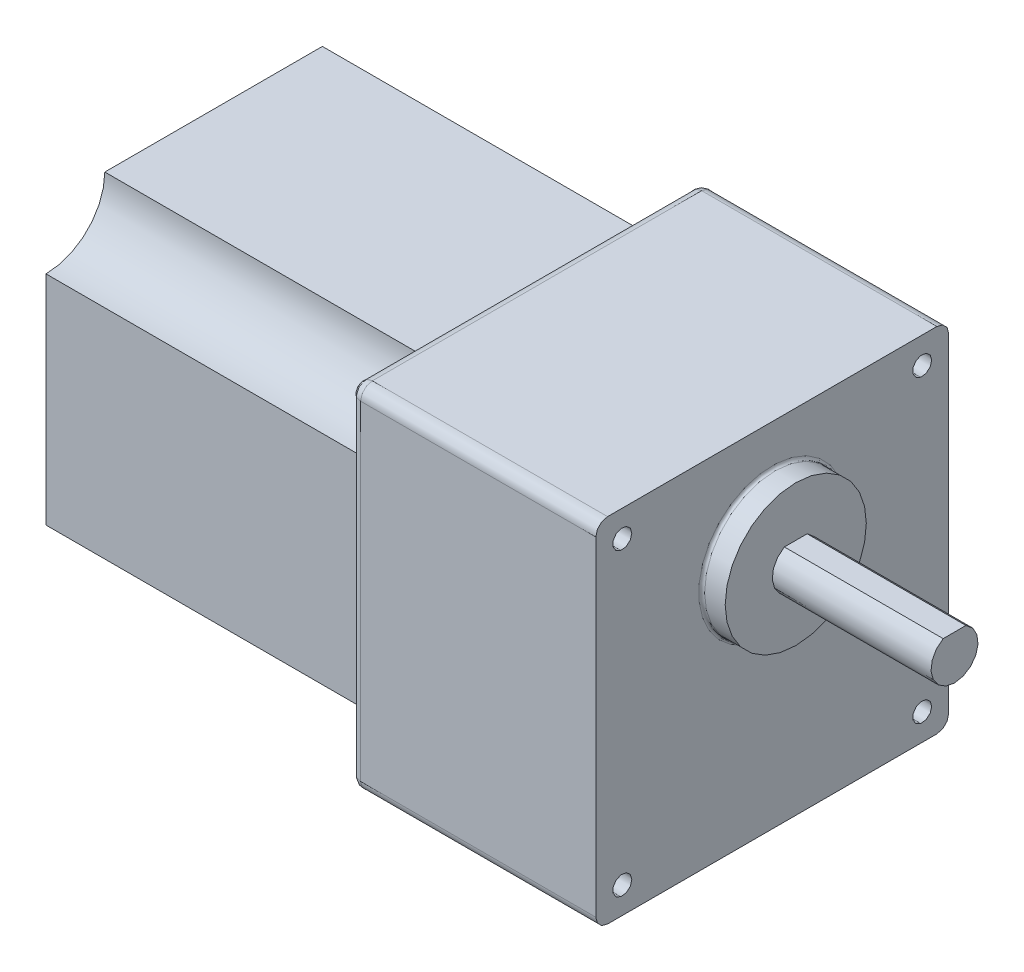
# Autodesk Inventor part: MOTOR MODEL
Saved by Autodesk Inventor 2023 (Build 270158000, 158)
## iProperties
Created: 2022-09-15
Part Number: MOTOR MODEL
Material: Acetal Resin, Black
Document SubType Name: Modeling
Designer: D.C. Eksteen
Density: 1.425 g/cm^3
Appearance: Smooth - Black
Author: D.C. Eksteen
Autodesk Inventor part; units mm, degrees
ref_plane "YZ Plane" through (0, 0, 0) normal (1, 0, 0) x (0, 1, 0)
ref_plane "XZ Plane" through (0, 0, 0) normal (0, 1, 0) x (-1, 0, 0)
ref_plane "XY Plane" through (0, 0, 0) normal (0, 0, 1) x (1, 0, 0)
sketch "Sketch1" plane through (0, 0, 0) normal (1, 0, 0) x (0, 1, 0)
  line L0 (0, 0) -> (60, 0)
  line L1 (60, 0) -> (60, -60)
  line L2 (60, -60) -> (0, -60)
  line L3 (0, -60) -> (0, 0)
  dimension "d0" = 60
  dimension "d1" = 60
  constraints: 8 end point, 2 parallel, 1 horizontal, 1 perpendicular
  measures "d0" distance of L1.end L2.end
  measures "d1" distance of L0.end L1.end
extrude "Extrusion1" add sketch "Sketch1" against normal blind 42
sketch "Sketch2" plane through (-42, 0, 0) normal (-1, 0, 0) x (0, 0, 1)
  line L0 (-60, 60) -> (-60, 0) projected
  line L1 (-60, 0) -> (0, 0) projected
  line L2 (0, 0) -> (0, 60) projected
  line L3 (0, 60) -> (-60, 60) projected
  line L4 (-58.5, 58.5) -> (-58.5, 1.5)
  line L5 (-58.5, 1.5) -> (-1.5, 1.5)
  line L6 (-1.5, 1.5) -> (-1.5, 58.5)
  line L7 (-1.5, 58.5) -> (-58.5, 58.5)
  dimension "d4" = 1.5
  constraints: 8 end point, 3 other
  measures "d4" distance between parallel lines of L3 L7
extrude "Extrusion2" add sketch "Sketch2" along normal blind 53 contours L7 L6 L5 L4
sketch "Sketch3" plane through (0, 0, 0) normal (1, 0, 0) x (0, 0, -1)
  line L0 (60, 0) -> (60, 60) projected
  line L1 (60, 60) -> (0, 60) projected
  line L2 (0, 60) -> (0, 0) projected
  line L3 (0, 0) -> (60, 0) projected
  circle A0 centre (30, 41) radius 12
  dimension "d8" = 24
  dimension "d9" = 19
  dimension "d10" = 30
  constraints: 1 centre point
  measures "d8" diameter of A0
  measures "d9" distance from line of L1 A0.centre
  measures "d10" distance from line of L2 A0.centre
extrude "Extrusion3" add sketch "Sketch3" along normal blind 4 contours A0
sketch "Sketch4" plane through (4, 41, -30) normal (1, 0, 0) x (0, 0, -1)
  circle A0 centre (0, 0) radius 12 projected
  circle A1 centre (0, 0) radius 4
  line L0 (-1.9365, 3.5) -> (1.9365, 3.5)
  point P0 (-30, -41)
  dimension "d13" = 8
  dimension "d16" = 3.5
  constraints: 2 end point, 2 point on circle, 1 centre point, 1 coincident, 1 horizontal
  measures "d13" diameter of A1
  measures "d16" distance from line of L0 A1.centre
extrude "Extrusion4" add sketch "Sketch4" along normal blind 27 contours A1 L0 picked at (0.0805, 0.6484)
sketch "Sketch5" plane through (0, 0, 0) normal (1, 0, 0) x (0, 0, -1)
  point P0 (0, 0)
sketch "Sketch6" plane through (-95, 0, 0) normal (-1, 0, 0) x (0, 0, 1)
  point P0 (0, 0)
fillet "Fillet2" radius 10 4 edges at (-68.5, 58.5, -58.5) (-68.5, 1.5, -58.5) (-68.5, 1.5, -1.5) (-68.5, 58.5, -1.5) inverted yes
fillet "Fillet3" radius 2 8 edges at (-42, 30, -60) (-42, 60, -30) (-21, 60, -60) (-42, 0, -30) (-21, 0, -60) (-21, 60, 0) (-42, 30, 0) (-21, 0, 0)
fillet "Fillet4" radius 0.5 1 edges at (0, 41, -18)
sketch "Sketch7" plane through (0, 0, 0) normal (1, 0, 0) x (0, 0, -1)
  arc A0 (0, 2) -> (2, 0) centre (2, 2) ccw projected
  line L0 (2, 0) -> (58, 0) projected
  arc A1 (58, 0) -> (60, 2) centre (58, 2) ccw projected
  line L1 (60, 2) -> (60, 58) projected
  arc A2 (60, 58) -> (58, 60) centre (58, 58) ccw projected
  line L2 (58, 60) -> (2, 60) projected
  arc A3 (2, 60) -> (0, 58) centre (2, 58) ccw projected
  line L3 (0, 58) -> (0, 2) projected
  circle A4 centre (30, 41) radius 12.5 projected
  line L4 (55.5, 55.5) -> (55.5, 4.5)
  line L5 (55.5, 4.5) -> (4.5, 4.5)
  line L6 (4.5, 4.5) -> (4.5, 55.5)
  line L7 (4.5, 55.5) -> (55.5, 55.5)
  point P0 (0, 0)
  dimension "d20" = 4.5
  constraints: 8 end point, 4 coincident, 3 other
  measures "d20" distance between parallel lines of L1 L4
hole "Hole1" at (0, 55.5, -55.5) at (0, 4.5, -55.5) at (0, 4.5, -4.5) at (0, 55.5, -4.5) direction (-1, 0, 0) diameter 3.242 end through all thread size "M4x0.7" class "6H" standard "ANSI Metric M Profile"
body "Solid1"
